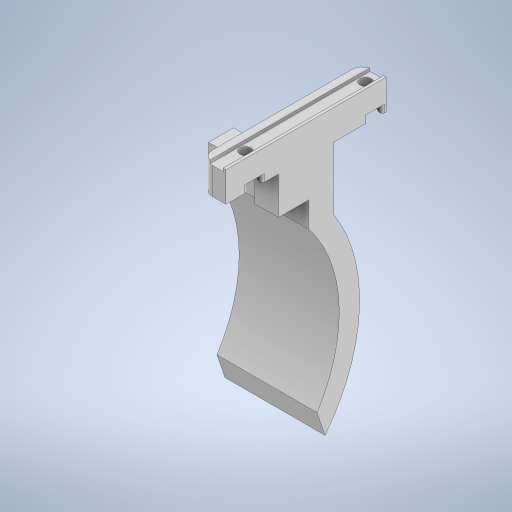
# Autodesk Inventor part: Back
Saved by Autodesk Inventor 2024 (Build 280153000, 153)
## iProperties
Created: 2023-12-18
Part Number: Back
Material: Generic
Document SubType Name: Modeling
Designer: Mechatronics Lab 1
Density: 1 g/cm^3
Appearance: Default
Author: Mechatronics Lab 1
Autodesk Inventor part; units mm, degrees
ref_plane "YZ Plane" through (0, 0, 0) normal (1, 0, 0) x (0, 1, 0)
ref_plane "XZ Plane" through (0, 0, 0) normal (0, 1, 0) x (-1, 0, 0)
ref_plane "XY Plane" through (0, 0, 0) normal (0, 0, 1) x (1, 0, 0)
sketch "Sketch1" plane through (0, 0, 0) normal (0, 1, 0) x (-1, 0, 0)
  line L0 (0, 0) -> (9.5, 0)
  line L1 (9.5, 0) -> (9.5, -64)
  line L2 (9.5, -64) -> (0, -64)
  line L3 (0, -64) -> (0, 0)
  circle A0 centre (3.7, -11.5) radius 2.25
  circle A1 centre (3.7, -59.5) radius 2.25
  line L4 (3.7, -11.5) -> (3.7, -59.5) construction
  dimension "d1" = 9.5
  dimension "d2" = 64
  dimension "d3" = 4.5
  dimension "d4" = 48
  dimension "d6" = 3.7
  dimension "d17" = 4.5
  constraints: 10 end point, 2 centre point, 2 parallel, 1 equal radius, 1 horizontal, 1 perpendicular, 1 vertical
  measures "d1" distance of L0.start L0.end
  measures "d2" distance of L0.end L1.end
  measures "d3" diameter of A0
  measures "d4" distance of L4.start L4.end
  measures "d6" distance between parallel lines of L3 L4
  measures "d17" distance from line of L4.end L2
extrude "Extrusion1" add sketch "Sketch1" along normal blind 12
sketch "Sketch2" plane through (-9.5, 0, 0) normal (0, 0, 1) x (1, 0, 0)
  line L0 (9.5, 12) -> (0, 12) projected
  line L1 (3, 12) -> (8.4, 12)
  line L2 (8.4, 12) -> (8.4, 10.8)
  line L3 (8.4, 10.8) -> (3, 10.8)
  line L4 (3, 10.8) -> (3, 12)
  line L5 (9.5, 0) -> (9.5, 12) projected
  line L6 (3.55, 0) -> (8.05, 0) projected
  line L7 (3.55, 12) -> (8.05, 12) projected
  line L8 (9.5, 0) -> (9.5, 12) projected
  line L9 (9.5, 0) -> (9.5, 12) projected
  line L10 (3.55, 12) -> (8.05, 12) projected
  line L11 (3.55, 12) -> (3.55, 0) projected
  line L12 (3.55, 12) -> (8.05, 12) projected
  line L13 (3.55, 0) -> (8.05, 0) projected
  line L14 (3.55, 12) -> (8.05, 12) projected
  line L15 (3.55, 0) -> (8.05, 0) projected
  line L16 (3.55, 12) -> (8.05, 12) projected
  line L17 (3.55, 0) -> (8.05, 0) projected
  dimension "d9" = 1.1
  dimension "d10" = 5.4
  dimension "d11" = 1.2
  dimension "d76" = 12
  constraints: 8 end point, 2 parallel, 1 horizontal, 1 perpendicular, 1 point on line
  measures "d9" distance between parallel lines of L5 L2
  measures "d10" distance of L2.end L3.end
  measures "d11" distance between parallel lines of L0 L3
  measures "d76" distance between parallel lines of L6 L7
extrude "Extrusion2" cut sketch "Sketch2" against normal up to next
sketch "Sketch3" plane through (0, 0, 0) normal (0, -1, 0) x (1, 0, 0)
  circle A0 centre (-3.7, -11.5) radius 2.25 projected
  circle A1 centre (-3.7, -11.5) radius 3.75
  circle A2 centre (-3.7, -59.5) radius 2.25 projected
  circle A3 centre (-3.7, -59.5) radius 3.75
  point P0 (0, 0)
  dimension "d14" = 7.5
  constraints: 2 centre point, 2 coincident, 1 equal radius
  measures "d14" diameter of A3
extrude "Extrusion3" cut sketch "Sketch3" against normal blind 3
fillet "Fillet1" radius 1 4 edges at (0, 1.5, -58.8897) (0, 1.5, -60.1103) (0, 1.5, -10.8897) (0, 1.5, -12.1103)
fillet "Fillet2" radius 4 2 edges at (-9.5, 6, -64) (-9.5, 6, 0)
sketch "Sketch15" plane through (0, 0, 0) normal (0, -1, 0) x (1, 0, 0)
  line L0 (0, 0) -> (0, -7.592) projected
  line L1 (-9.5, -32) -> (-9.5, -21)
  line L2 (-9.5, -21) -> (0, -21)
  line L3 (0, -21) -> (0, -43)
  line L4 (0, -43) -> (-9.5, -43)
  line L5 (-9.5, -43) -> (-9.5, -32)
  dimension "d79" = 11
  dimension "d80" = 22
  constraints: 10 end point, 2 perpendicular
  measures "d79" distance of L1.start L1.end
  measures "d80" distance of L2.end L3.end
extrude "Extrusion15" add sketch "Sketch15" along normal blind 15
sketch "Sketch16" plane through (0, -15, 0) normal (0, -1, 0) x (1, 0, 0)
  line L0 (0, -43) -> (-9.5, -43) projected
  line L1 (0, -43) -> (-40, -43)
  line L2 (-40, -43) -> (-40, -33)
  line L3 (-40, -33) -> (0, -33)
  line L4 (0, -33) -> (0, -43)
  point P0 (0, 0)
  dimension "d83" = 40
  dimension "d84" = 10
  constraints: 8 end point, 2 parallel, 1 horizontal, 1 perpendicular
  measures "d83" distance of L2.end L3.end
  measures "d84" distance of L1.end L2.end
extrude "Extrusion16" add sketch "Sketch16" along normal blind 10
sketch "Sketch17" plane through (0, -25, 0) normal (0, -1, 0) x (1, 0, 0)
  line L0 (0, -33) -> (0, -21) projected
  line L1 (-40, -43) -> (-9.5, -43) projected
  line L2 (0, -33) -> (-40, -33)
  line L3 (-40, -33) -> (-40, -43)
  line L4 (-40, -43) -> (0, -43)
  line L5 (0, -43) -> (0, -33)
  point P0 (0, 0)
  point P1 (-9.5, -43)
  constraints: 8 end point, 2 parallel, 1 horizontal, 1 perpendicular
sketch "Sketch18" plane through (-40, -15, -43) normal (-1, 0, 0) x (0, 0, 1)
  line L0 (0, -10) -> (10, -10) projected
  arc A0 (5, -10) -> (5, -80) centre (53.734, -45) ccw
  point P0 (43, 15)
  dimension "d87" = 70
  dimension "d88" = 60
  constraints: 2 point on circle, 1 centre point, 1 midpoint
  measures "d87" distance of A0.start A0.end
  measures "d88" radius of A0
sweep "Sweep1" add profiles "Sketch17" path "Sketch18" path curves A0
body "Solid1"
